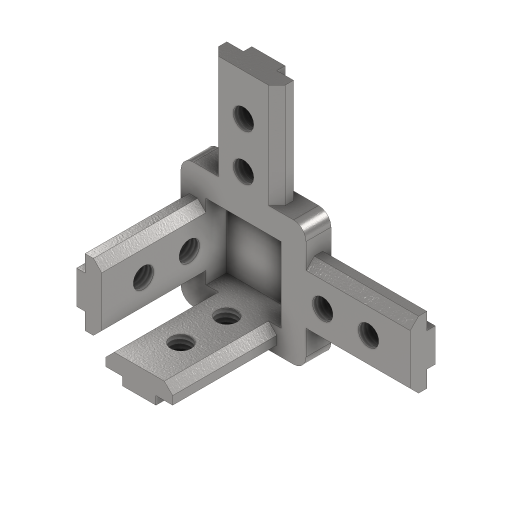
# Autodesk Inventor part: Sambungan Siku
Saved by Autodesk Inventor 2024.4 (Build 284460000, 460)
## iProperties
Created: 2025-10-20
Part Number: Sambungan Siku
Material: Generic
Document SubType Name: Modeling
Designer: Hp
Density: 1 g/cm^3
Appearance: Galvanized
Author: Hp
Autodesk Inventor part; units mm, degrees
sketch "Sketch1" plane through (0, 0, 0) normal (0, 0, 1) x (1, 0, 0)
  line L0 (15, -15) -> (-15, -15)
  line L1 (-15, -15) -> (-15, 15)
  line L2 (-15, 15) -> (15, 15)
  line L3 (15, 15) -> (15, -15)
  line L4 (15, -15) -> (-15, 15) construction
  line L5 (-15, -15) -> (15, 15) construction
  point P0 (0, 0)
  dimension "d0" = 30
  dimension "d1" = 30
  constraints: 12 end point, 2 midpoint, 2 parallel, 1 horizontal, 1 perpendicular
  measures "d0" distance of L1.end L2.end
  measures "d1" distance of L2.end L0.start
extrude "Extrusion1" add sketch "Sketch1" along normal blind 6
sketch "Sketch7" plane through (0, 0, 6) normal (0, 0, 1) x (1, 0, 0)
  line L0 (9, -9) -> (-9, -9)
  line L1 (-9, -9) -> (-9, 9)
  line L2 (-9, 9) -> (9, 9)
  line L3 (9, 9) -> (9, -9)
  line L4 (9, -9) -> (-9, 9) construction
  line L5 (-9, -9) -> (9, 9) construction
  line L6 (15, -15) -> (15, 15) projected
  line L7 (15, 15) -> (-15, 15) projected
  point P0 (0, 0)
  dimension "d59" = 6
  dimension "d60" = 6
  constraints: 12 end point, 2 midpoint, 2 parallel, 1 horizontal, 1 perpendicular
  measures "d59" distance between parallel lines of L6 L3
  measures "d60" distance between parallel lines of L7 L2
extrude "Extrusion5" cut sketch "Sketch7" against normal blind 5
sketch "Sketch2" plane through (-10, 10, 1) normal (0, 0, 1) x (1, 0, 0)
  line L0 (14, -25) -> (6, -25)
  line L1 (2, -23) -> (18, -23)
  line L2 (-5, -25) -> (25, -25) projected
  line L3 (2, -23) -> (2, -21)
  line L4 (2, -21) -> (4, -19)
  line L5 (4, -19) -> (16, -19)
  line L6 (16, -19) -> (18, -21)
  line L7 (18, -21) -> (18, -23)
  line L8 (6, -23) -> (6, -25)
  line L9 (14, -25) -> (14, -23)
  point P0 (10, -10)
  point P1 (10, -25)
  point P2 (10, -25)
  point P3 (10, -19)
  point P4 (10, -25)
  point P5 (10, -23)
  dimension "d6" = 12
  dimension "d7" = 8
  dimension "d9" = 16
  dimension "d10" = 4
  dimension "d11" = 2
  dimension "d26" = 8
  dimension "d27" = 45
  dimension "d63" = 6
  constraints: 18 end point, 5 midpoint, 4 point on line, 2 equal length, 2 horizontal, 2 perpendicular, 2 vertical alignment, 1 coincident, 1 collinear, 1 parallel, 1 vertical
  measures "d6" distance of L4.end L5.end
  measures "d7" distance between parallel lines of L8 L9
  measures "d9" distance of L1.start L1.end
  measures "d10" distance between parallel lines of L1 L5
  measures "d11" distance of L6.end L1.end
  measures "d26" distance from line of point (10, -10) L7
  measures "d27" angle of L7 L6
  measures "d63" distance between parallel lines of L5 L0
extrude "Extrusion2" add sketch "Sketch2" along normal blind 25 from surface at 5
ref_plane "Work Plane3" through (-6, -5, 5) normal (0, 1, 0) x (1, 0, 0)
sketch "Sketch3" plane through (-6, -9, 5) normal (0, 1, 0) x (1, 0, 0)
  circle A0 centre (6, -16) radius 3
  line L0 (6, -16) -> (6, -5) construction
  line L1 (0, -26) -> (12, -26) construction
  circle A1 centre (6, -5) radius 3
  point P0 (6, 5)
  point P1 (6, -26)
  point P2 (6, -26)
  dimension "d16" = 6
  dimension "d65" = 11
  dimension "d66" = 10
  constraints: 3 coincident, 2 centre point, 2 end point, 1 equal radius, 1 midpoint, 1 vertical, 1 vertical alignment
  measures "d16" diameter of A0
  measures "d65" distance of L0.start L0.end
  measures "d66" distance of point (6, -26) L0.start
hole "Hole1" at (0, -9, 21) at (0, -9, 10) direction (0, -1, 0) diameter 4.917 end through all thread size "M6x1" class "6H" standard "ANSI Metric M Profile"
ref_plane "Work Plane1" through (-15, -15, 0) normal (-0.7071068, 0.7071068, 0) x (0, 0, -1)
sketch "Sketch4" plane through (-15, 15, 0) normal (0, 1, 0) x (1, 0, 0)
  line L0 (11, 0) -> (19, 0)
  line L1 (23, -2) -> (7, -2)
  line L2 (23, -2) -> (23, -4)
  line L3 (23, -4) -> (21, -6)
  line L4 (21, -6) -> (9, -6)
  line L5 (9, -6) -> (7, -4)
  line L6 (7, -4) -> (7, -2)
  line L7 (19, -2) -> (19, 0)
  line L8 (11, 0) -> (11, -2)
  line L9 (30, 0) -> (0, 0) construction
  line L10 (30, -6) -> (0, -6) construction
  point P0 (15, 0)
  point P1 (15, -6)
  point P2 (15, 0)
  point P3 (15, -2)
  point P4 (15, -6)
  point P5 (15, 0)
  point P6 (15, 0)
  point P7 (15, -6)
  point P8 (15, 0)
  dimension "d28" = 12
  dimension "d29" = 8
  dimension "d30" = 16
  dimension "d31" = 4
  dimension "d32" = 2
  dimension "d34" = 45
  constraints: 18 end point, 8 midpoint, 3 parallel, 3 vertical alignment, 2 coincident, 2 equal length, 2 perpendicular, 2 point on line
  measures "d28" distance of L4.start L5.start
  measures "d29" distance between parallel lines of L7 L8
  measures "d30" distance of L2.start L1.end
  measures "d31" distance between parallel lines of L1 L4
  measures "d32" distance of L5.end L1.end
  measures "d34" angle of L6 L5
extrude "Extrusion3" add sketch "Sketch4" along normal blind 25
sketch "Sketch5" plane through (0, 0, 6) normal (0, 0, 1) x (1, 0, 0)
  line L0 (0, 30) -> (0, 19) construction
  line L1 (-6, 40) -> (6, 40) construction
  point P0 (0, 0)
  point P1 (0, 40)
  dimension "d41" = 10
  dimension "d42" = 11
  constraints: 2 end point, 1 midpoint, 1 vertical, 1 vertical alignment
  measures "d41" distance from line of L1 L0.start
  measures "d42" distance of L0.start L0.end
hole "Hole2" at (0, 19, 6) at (0, 30, 6) direction (0, 0, -1) diameter 4.917 end through all thread size "M6x1" class "6H" standard "ANSI Metric M Profile"
mirror "Mirror2" about plane through (-15, -15, 0) normal (-0.7071068, 0.7071068, 0) of "Hole2", "Extrusion3"
ref_plane "Work Plane2" through (-10, 10, 5) normal (0, 0, 1) x (1, 0, 0)
fillet "Fillet1" radius 3 4 edges at (15, 15, 3) (-15, 15, 3) (-15, -15, 3) (15, -15, 3)
mirror "Mirror3" about plane through (-15, -15, 0) normal (-0.7071068, 0.7071068, 0) of "Hole1", "Extrusion2"
equation "\"d1\" = d0"
equation "\"d60\" = d59"
equation "\"d26\" = 0.5 * d9"
body "Solid1"
